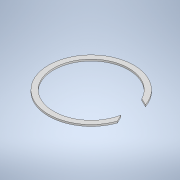
# Autodesk Inventor part: 79. Кольцо стопорное
Saved by Autodesk Inventor 2021 (Build 250183000, 183)
## iProperties
Created: 2021-03-15
Part Number: 79. Кольцо стопорное
Material: Типовые
Document SubType Name: Modeling
Designer: Данил
Density: 1 g/cm^3
Appearance: По умолчанию
Author: Данил
Autodesk Inventor part; units mm, degrees
ref_plane "YZ Plane" through (0, 0, 0) normal (1, 0, 0) x (0, 1, 0)
ref_plane "XZ Plane" through (0, 0, 0) normal (0, 1, 0) x (-1, 0, 0)
ref_plane "XY Plane" through (0, 0, 0) normal (0, 0, 1) x (1, 0, 0)
sketch "Эскиз1" plane through (0, 0, 0) normal (0, 0, 1) x (1, 0, 0)
  line L0 (0, 0.85) -> (0, -0.85)
  line L1 (38, 0.85) -> (43.2, 0.85)
  line L2 (43.2, 0.85) -> (43.2, -0.85)
  line L3 (43.2, -0.85) -> (38, -0.85)
  line L4 (38, -0.85) -> (38, 0.85)
  point P0 (0, 0)
  point P1 (0, 0)
  dimension "d0" = 1.7
  dimension "d1" = 86.4
  dimension "d2" = 76
  constraints: 10 end point, 2 horizontal alignment, 2 parallel, 1 coincident, 1 horizontal, 1 midpoint, 1 perpendicular, 1 vertical
  measures "d0" distance of L0.start L0.end
  measures "d1" diameter of L2 L0
  measures "d2" diameter of L4 L0
revolve "Вращение1" add sketch "Эскиз1" angle 360 about axis through (0, 0.85, 0) along (0, -1, 0)
sketch "Эскиз2" plane through (0, 0.85, 0) normal (0, 1, 0) x (1, 0, 0)
  line L0 (40.7646, 14.3) -> (40.7646, -14.3)
  circle A0 centre (0, 0) radius 43.2 projected
  line L1 (0, 0) -> (40.7646, 14.3)
  line L2 (40.7646, 14.3) -> (0, 33.8918)
  circle A1 centre (0, 0) radius 38 projected
  line L3 (0, 0) -> (40.7646, -14.3)
  line L4 (40.7646, -14.3) -> (29.0022, 10.1738)
  point P0 (0, 0)
  point P1 (40.7646, 0)
  point P2 (33.6042, 17.7413)
  point P3 (35.8577, 12.5787)
  dimension "d4" = 28.6
  dimension "d5" = 45
  dimension "d6" = 45
  constraints: 10 end point, 1 horizontal alignment, 1 midpoint, 1 point on line, 1 vertical, 1 vertical alignment, 2 other
  measures "d4" distance of L0.start L0.end
  measures "d5" angle of L1 L2
  measures "d6" angle of L3 L4
extrude "Выдавливание1" cut sketch "Эскиз2" against normal through all contours A0 L0 | L0 L4 A1 L1 | L1 A1 L2 | A1 L4 L1
